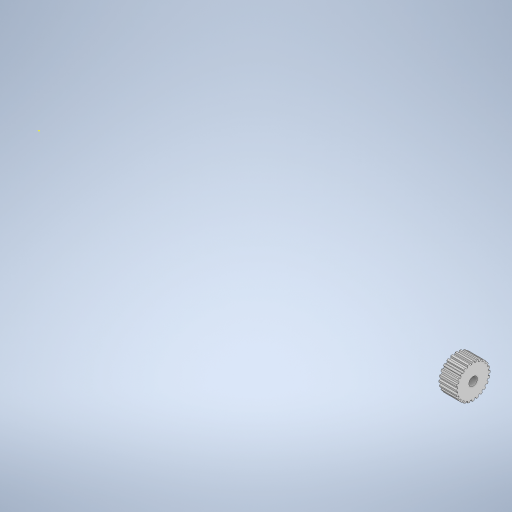
# Autodesk Inventor part: parte adicional
Saved by Autodesk Inventor 2024 (Build 280153000, 153)
## iProperties
Created: 2024-03-31
Part Number: parte adicional
Material: Generic
Document SubType Name: Modeling
Designer: menes
Density: 1 g/cm^3
Appearance: Default
Author: menes
Autodesk Inventor part; units mm, degrees
ref_plane "Work Plane1" through (254, 0, 0) normal (1, 0, 0) x (0, 0, -1)
ref_plane "Work Plane2" through (254, 0, 0) normal (1, 0, 0) x (0, 0, -1)
sketch "Sketch3" plane through (254, 0, 0) normal (1, 0, 0) x (0, 0, -1)
  arc A0 (-0.5014, 9.9874) -> (0.4986, 9.9876) centre (0, 0) ccw
  line L0 (0.4986, 9.9876) -> (-0.5014, 9.9874)
  line L1 (-0.5014, 9.9874) -> (-0.7511, 8.9686)
  line L2 (0.4986, 9.9876) -> (0.7489, 8.9688)
  line L3 (-3.0693, 9.5173) -> (-3.0468, 8.4686)
  line L4 (-2.1034, 9.7763) -> (-3.0693, 9.5173)
  line L5 (-2.1034, 9.7763) -> (-1.5979, 8.857)
  line L6 (-5.428, 8.3986) -> (-5.1348, 7.3915)
  line L7 (-4.562, 8.8988) -> (-5.428, 8.3986)
  line L8 (-4.562, 8.8988) -> (-3.8358, 8.1416)
  line L9 (-7.4167, 6.7076) -> (-6.8729, 5.8106)
  line L10 (-6.7097, 7.4148) -> (-7.4167, 6.7076)
  line L11 (-6.7097, 7.4148) -> (-5.8124, 6.8714)
  line L12 (-8.9001, 4.5595) -> (-8.1426, 3.8338)
  line L13 (-8.4002, 5.4256) -> (-8.9001, 4.5595)
  line L14 (-8.4002, 5.4256) -> (-7.3928, 5.1329)
  line L15 (-9.7769, 2.1006) -> (-8.8574, 1.5957)
  line L16 (-9.5182, 3.0666) -> (-9.7769, 2.1006)
  line L17 (-9.5182, 3.0666) -> (-8.4694, 3.0447)
  line L18 (-9.9874, -0.5014) -> (-8.9686, -0.7511)
  line L19 (-9.9876, 0.4986) -> (-9.9874, -0.5014)
  line L20 (-9.9876, 0.4986) -> (-8.9688, 0.7489)
  line L21 (-9.5173, -3.0693) -> (-8.4686, -3.0468)
  line L22 (-9.7763, -2.1034) -> (-9.5173, -3.0693)
  line L23 (-9.7763, -2.1034) -> (-8.857, -1.5979)
  line L24 (-8.3986, -5.428) -> (-7.3915, -5.1348)
  line L25 (-8.8988, -4.562) -> (-8.3986, -5.428)
  line L26 (-8.8988, -4.562) -> (-8.1416, -3.8358)
  line L27 (-6.7076, -7.4167) -> (-5.8106, -6.8729)
  line L28 (-7.4148, -6.7097) -> (-6.7076, -7.4167)
  line L29 (-7.4148, -6.7097) -> (-6.8714, -5.8124)
  line L30 (-4.5595, -8.9001) -> (-3.8338, -8.1426)
  line L31 (-5.4256, -8.4002) -> (-4.5595, -8.9001)
  line L32 (-5.4256, -8.4002) -> (-5.1329, -7.3928)
  line L33 (-2.1006, -9.7769) -> (-1.5957, -8.8574)
  line L34 (-3.0666, -9.5182) -> (-2.1006, -9.7769)
  line L35 (-3.0666, -9.5182) -> (-3.0447, -8.4694)
  line L36 (0.5014, -9.9874) -> (0.7511, -8.9686)
  line L37 (-0.4986, -9.9876) -> (0.5014, -9.9874)
  line L38 (-0.4986, -9.9876) -> (-0.7489, -8.9688)
  line L39 (3.0693, -9.5173) -> (3.0468, -8.4686)
  line L40 (2.1034, -9.7763) -> (3.0693, -9.5173)
  line L41 (2.1034, -9.7763) -> (1.5979, -8.857)
  line L42 (5.428, -8.3986) -> (5.1348, -7.3915)
  line L43 (4.562, -8.8988) -> (5.428, -8.3986)
  line L44 (4.562, -8.8988) -> (3.8358, -8.1416)
  line L45 (7.4167, -6.7076) -> (6.8729, -5.8106)
  line L46 (6.7097, -7.4148) -> (7.4167, -6.7076)
  line L47 (6.7097, -7.4148) -> (5.8124, -6.8714)
  line L48 (8.9001, -4.5595) -> (8.1426, -3.8338)
  line L49 (8.4002, -5.4256) -> (8.9001, -4.5595)
  line L50 (8.4002, -5.4256) -> (7.3928, -5.1329)
  line L51 (9.7769, -2.1006) -> (8.8574, -1.5957)
  line L52 (9.5182, -3.0666) -> (9.7769, -2.1006)
  line L53 (9.5182, -3.0666) -> (8.4694, -3.0447)
  line L54 (9.9874, 0.5014) -> (8.9686, 0.7511)
  line L55 (9.9876, -0.4986) -> (9.9874, 0.5014)
  line L56 (9.9876, -0.4986) -> (8.9688, -0.7489)
  line L57 (9.5173, 3.0693) -> (8.4686, 3.0468)
  line L58 (9.7763, 2.1034) -> (9.5173, 3.0693)
  line L59 (9.7763, 2.1034) -> (8.857, 1.5979)
  line L60 (8.3986, 5.428) -> (7.3915, 5.1348)
  line L61 (8.8988, 4.562) -> (8.3986, 5.428)
  line L62 (8.8988, 4.562) -> (8.1416, 3.8358)
  line L63 (6.7076, 7.4167) -> (5.8106, 6.8729)
  line L64 (7.4148, 6.7097) -> (6.7076, 7.4167)
  line L65 (7.4148, 6.7097) -> (6.8714, 5.8124)
  line L66 (4.5595, 8.9001) -> (3.8338, 8.1426)
  line L67 (5.4256, 8.4002) -> (4.5595, 8.9001)
  line L68 (5.4256, 8.4002) -> (5.1329, 7.3928)
  line L69 (2.1006, 9.7769) -> (1.5957, 8.8574)
  line L70 (3.0666, 9.5182) -> (2.1006, 9.7769)
  line L71 (3.0666, 9.5182) -> (3.0447, 8.4694)
  arc A1 (-0.7511, 8.9686) -> (-1.5979, 8.857) centre (0, 0) ccw
  arc A2 (-3.0468, 8.4686) -> (-3.8358, 8.1416) centre (0, 0) ccw
  arc A3 (-5.1348, 7.3915) -> (-5.8124, 6.8714) centre (0, 0) ccw
  arc A4 (-6.8729, 5.8106) -> (-7.3928, 5.1329) centre (0, 0) ccw
  arc A5 (-8.1426, 3.8338) -> (-8.4694, 3.0447) centre (0, 0) ccw
  arc A6 (-8.8574, 1.5957) -> (-8.9688, 0.7489) centre (0, 0) ccw
  arc A7 (-8.9686, -0.7511) -> (-8.857, -1.5979) centre (0, 0) ccw
  arc A8 (-8.4686, -3.0468) -> (-8.1416, -3.8358) centre (0, 0) ccw
  arc A9 (-7.3915, -5.1348) -> (-6.8714, -5.8124) centre (0, 0) ccw
  arc A10 (-5.8106, -6.8729) -> (-5.1329, -7.3928) centre (0, 0) ccw
  arc A11 (-3.8338, -8.1426) -> (-3.0447, -8.4694) centre (0, 0) ccw
  arc A12 (-1.5957, -8.8574) -> (-0.7489, -8.9688) centre (0, 0) ccw
  arc A13 (0.7511, -8.9686) -> (1.5979, -8.857) centre (0, 0) ccw
  arc A14 (3.0468, -8.4686) -> (3.8358, -8.1416) centre (0, 0) ccw
  arc A15 (5.1348, -7.3915) -> (5.8124, -6.8714) centre (0, 0) ccw
  arc A16 (6.8729, -5.8106) -> (7.3928, -5.1329) centre (0, 0) ccw
  arc A17 (8.1426, -3.8338) -> (8.4694, -3.0447) centre (0, 0) ccw
  arc A18 (8.8574, -1.5957) -> (8.9688, -0.7489) centre (0, 0) ccw
  arc A19 (8.9686, 0.7511) -> (8.857, 1.5979) centre (0, 0) ccw
  arc A20 (8.4686, 3.0468) -> (8.1416, 3.8358) centre (0, 0) ccw
  arc A21 (7.3915, 5.1348) -> (6.8714, 5.8124) centre (0, 0) ccw
  arc A22 (5.8106, 6.8729) -> (5.1329, 7.3928) centre (0, 0) ccw
  arc A23 (3.8338, 8.1426) -> (3.0447, 8.4694) centre (0, 0) ccw
  arc A24 (1.5957, 8.8574) -> (0.7489, 8.9688) centre (0, 0) ccw
  dimension "d24" = 1.5
  dimension "d25" = 1
  dimension "d28" = 360
  constraints: 144 end point, 50 point on circle, 25 centre point, 2 coincident, 169 other
  measures "d24" distance of L2.end L1.end
  measures "d25" distance of L0.start L0.end
extrude "Extrusion3" add sketch "Sketch3" against normal blind 10 contours L0 L2 A24 L69 L70 L71 A23 L66 L67 L68 A22 L63 L64 L65 A21 L60 L61 L62 A20 L57 L58 L59 A19 L54 L55 L56 A18 L51 L52 L53 A17 L48 L49 L50 A16 L45 L46 L47 A15 L42 L43 L44 A14 L39 L40 L41 A13 L36 L37 L38 A12 L33 L34 L35 A11 L30 L31 L32 A10 L27 L28 L29 A9 L24 L25 L26 A8 L21 L22 L23 A7 L18 L19 L20 A6 L15 L16 L17 A5 L12 L13 L14 A4 L9 L10 L11 A3 L6 L7 L8 A2 L3 L4 L5 A1 L1
ref_plane "Work Plane3" through (254, 0, 0) normal (1, 0, 0) x (0, 0, -1)
sketch "Sketch4" plane through (254, 0, 0) normal (1, 0, 0) x (0, 0, -1)
  circle A0 centre (0, 0) radius 2.5
  dimension "d32" = 5
  constraints: 1 centre point, 1 coincident
  measures "d32" diameter of A0
extrude "Extrusion4" cut sketch "Sketch4" against normal blind 10
sketch "Sketch5" plane through (0, 0, 0) normal (1, 0, 0) x (0, 1, 0)
  point P0 (0, 0)
body "Solid1"
